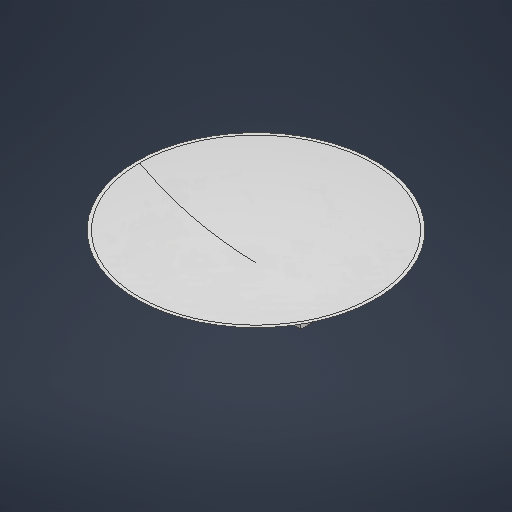
# Autodesk Inventor part: ensayo9
Saved by Autodesk Inventor 2026.2 (Build 302298000, 298)
## iProperties
Created: 2025-12-22
Part Number: ensayo9
Material: Genérico
Document SubType Name: Modeling
Designer: vicho
Density: 1 g/cm^3
Appearance: Valor por defecto
Author: vicho
Autodesk Inventor part; units mm, degrees
ref_plane "YZ Plane" through (0, 0, 0) normal (1, 0, 0) x (0, 1, 0)
ref_plane "XY Plane" through (0, 0, 0) normal (0, 0, 1) x (1, 0, 0)
sketch "Boceto1" plane through (0, 0, 0) normal (0, 0, 1) x (1, 0, 0)
  line L0 (0, 50) -> (0, -50) construction
  line L1 (-50, 0) -> (50, 0) construction
  line L2 (-93.996, 20) -> (36.7723, 20) construction
  line L3 (-80, 55.4649) -> (-80, -15.4649) construction
  spline S0 degree 2 poles (-80, 20) (-46.298, 1.0518) (0, 0) knots 0 0 0 1 1 1
  line L4 (0, 20) -> (-80, 20)
  line L5 (0, 20) -> (0, 0)
  point P0 (-45, 6)
  dimension "d0" = 100
  dimension "d1" = 100
  dimension "d2" = 20
  dimension "d3" = 80
  dimension "d4" = 14
  dimension "d5" = 45
  dimension "d6" = 36.7723
  dimension "d7" = 55.4649
  dimension "d8" = 93.996
  constraints: 12 end point, 3 midpoint, 2 collinear, 2 horizontal, 2 point on line, 2 symmetric about line, 2 vertical, 3 other
  measures "d0" distance of L1.end L1.start
  measures "d1" distance of L0.end L0.start
  measures "d2" distance between parallel lines of L1 L2
  measures "d3" distance between parallel lines of L3 L0
  measures "d4" distance from line of point (-45, 6) L2
  measures "d5" distance from line of point (-45, 6) L0
  measures "d6" distance from line of L2.end L0
  measures "d7" distance from line of L3.start L1
  measures "d8" distance from line of L2.start L0
revolve "Revolución1" add sketch "Boceto1" angle 360 about axis through (0, 20, 0) along (0, -1, 0)
shell "Vaciado1" thickness 1 removed faces 1 at (-23.7602, 20, 12.1064)
ref_plane "Plano de trabajo1" through (0, -10, 0) normal (0, 1, 0) x (-1, 0, 0)
sketch "Boceto2" plane through (0, -10, 0) normal (0, 1, 0) x (-1, 0, 0)
  line L0 (-42.5, -12.5) -> (-27.5, -12.5)
  line L1 (-27.5, -12.5) -> (-27.5, 12.5)
  line L2 (-27.5, 12.5) -> (-42.5, 12.5)
  line L3 (-42.5, 12.5) -> (-42.5, -12.5)
  line L4 (-42.5, -12.5) -> (-27.5, 12.5) construction
  line L5 (-27.5, -12.5) -> (-42.5, 12.5) construction
  line L6 (27.5, -12.5) -> (42.5, -12.5)
  line L7 (42.5, -12.5) -> (42.5, 12.5)
  line L8 (42.5, 12.5) -> (27.5, 12.5)
  line L9 (27.5, 12.5) -> (27.5, -12.5)
  line L10 (27.5, -12.5) -> (42.5, 12.5) construction
  line L11 (42.5, -12.5) -> (27.5, 12.5) construction
  circle A0 centre (0, 0) radius 80 construction
  line L12 (0, 80) -> (0, -80) construction
  line L13 (76.5933, 0) -> (-80, 0) construction
  point P0 (-35, 0)
  point P1 (35, 0)
  point P2 (80, 0)
  dimension "d12" = 35
  dimension "d13" = 35
  dimension "d14" = 15
  dimension "d15" = 25
  dimension "d16" = 15
  dimension "d17" = 25
  dimension "d18" = 76.5933
  constraints: 28 end point, 4 horizontal, 4 midpoint, 4 parallel, 3 point on circle, 2 perpendicular, 2 vertical, 1 point on line, 1 other
  measures "d12" distance of point (0, 0) point (-35, 0)
  measures "d13" distance of point (0, 0) point (35, 0)
  measures "d14" distance of L1.end L2.end
  measures "d15" distance of L2.end L0.start
  measures "d16" distance of L7.end L8.end
  measures "d17" distance of L6.end L7.end
  measures "d18" distance from line of L13.start L12
extrude "Extrusión1" add sketch "Boceto2" along normal up to next
sketch "Boceto3" plane through (42.5, -10, 12.5) normal (1, 0, 0) x (0, 0, -1)
  line L0 (12.5, 97.2101) -> (12.5, -82.1758) construction
  line L1 (-112.7287, 7.5172) -> (171.2472, 7.5172) construction
  line L2 (0, 0) -> (25, 0) construction
  line L3 (25, 0) -> (25, 15.8181) construction
  point P0 (12.5, 10)
  point P1 (12.5, 7.5)
  dimension "d21" = 7.5
  dimension "d22" = 12.5
  constraints: 4 end point, 2 horizontal, 2 vertical, 1 point on line
  measures "d21" distance from line of L2 point (12.5, 7.5)
  measures "d22" distance from line of L3 point (12.5, 7.5)
hole "Agujero1" at (42.5, -2.5, 0) direction (-1, 0, 0) diameter 3 end through all countersink diameter 5 countersink angle 90
mirror "Simetría1" about plane through (0, 0, 0) normal (1, 0, 0) of "Agujero1"
